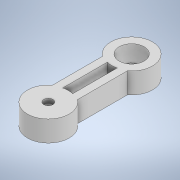
# Autodesk Inventor part: ramię_korby
Saved by Autodesk Inventor 2020 (Build 240168000, 168)
## iProperties
Created: 2020-08-09
Part Number: ramię_korby
Material: Aluminum 6061
Document SubType Name: Modeling
Designer: Hesekiel
Density: 2.7 g/cm^3
Appearance: Aluminum - Flat
Author: Hesekiel
Autodesk Inventor part; units mm, degrees
ref_plane "YZ Plane" through (0, 0, 0) normal (1, 0, 0) x (0, 1, 0)
ref_plane "XZ Plane" through (0, 0, 0) normal (0, 1, 0) x (-1, 0, 0)
ref_plane "XY Plane" through (0, 0, 0) normal (0, 0, 1) x (1, 0, 0)
sketch "Sketch1" plane through (0, 0, 0) normal (0, 1, 0) x (-1, 0, 0)
  circle A0 centre (0, 0) radius 15
  line L0 (15, 0) -> (-15, 0)
  line L1 (-15, 0) -> (-15, -100)
  line L2 (-15, -100) -> (15, -100)
  line L3 (15, -100) -> (15, 0)
  circle A1 centre (0, -100) radius 15
  circle A2 centre (0, 0) radius 25
  circle A3 centre (0, -100) radius 25
  point P0 (-15, -20)
  point P1 (-15, -80)
  point P2 (15, -80)
  point P3 (15, -20)
  dimension "d0" = 30
  dimension "d1" = 30
  dimension "d2" = 100
  dimension "d3" = 30
  dimension "d4" = 50
  dimension "d5" = 50
  constraints: 8 end point, 3 centre point, 3 coincident, 2 parallel, 1 horizontal, 1 horizontal alignment, 1 midpoint, 1 perpendicular, 2 other
  measures "d1" distance of L2.end L1.end
  measures "d2" distance of L1.end L0.end
  measures "d3" diameter of A1
  measures "d4" diameter of A2
  measures "d5" diameter of A3
extrude "Extrusion1" add sketch "Sketch1" along normal blind 15 contours L3 A2 L1 A0 | A0 L1 A2 L3 | L3 A3 L1 A2 | A3 L1 A1 L3 | L3 A1 L1 A3
shell "Shell1" thickness 9 removed faces 1 at (5, 15, -40)
sketch "Sketch2" plane through (0, 9, 0) normal (0, 1, 0) x (1, 0, 0)
  line L0 (-6, 76.7621) -> (-6, 23.2379) projected
  arc A0 (6, 23.2379) -> (-6, 23.2379) centre (0, 0) ccw projected
  line L1 (6, 23.2379) -> (6, 76.7621) projected
  arc A1 (-6, 76.7621) -> (6, 76.7621) centre (0, 100) ccw projected
extrude "Extrusion2" cut sketch "Sketch2" against normal blind 73.75
sketch "Sketch3" plane through (0, 0, 0) normal (0, -1, 0) x (1, 0, 0)
  line L0 (-6, -76.7621) -> (-6, -23.2379) projected
  arc A0 (-6, -23.2379) -> (6, -23.2379) centre (0, 0) ccw projected
  line L1 (6, -23.2379) -> (6, -76.7621) projected
  arc A1 (6, -76.7621) -> (-6, -76.7621) centre (0, -100) ccw projected
  arc A2 (-15, -80) -> (15, -80) centre (0, -100) ccw projected
  line L2 (15, -20) -> (15, -80) projected
  arc A3 (15, -20) -> (-15, -20) centre (0, 0) ccw projected
  line L3 (-15, -80) -> (-15, -20) projected
  circle A4 centre (0, 0) radius 15 projected
  circle A5 centre (0, -100) radius 15 projected
extrude "Extrusion3" add sketch "Sketch3" along normal blind 10
sketch "Sketch4" plane through (0, 15, 0) normal (0, 1, 0) x (1, 0, 0)
  circle A0 centre (0, 0) radius 15
  constraints: 1 centre point, 1 coincident
extrude "Extrusion4" add sketch "Sketch4" against normal blind 5
sketch "Sketch5" plane through (0, 15, 0) normal (0, 1, 0) x (1, 0, 0)
  circle A0 centre (0, 0) radius 5.5
  dimension "d15" = 11
  constraints: 1 centre point, 1 coincident
  measures "d15" diameter of A0
extrude "Extrusion5" cut sketch "Sketch5" against normal blind 89
sketch "Sketch6" plane through (0, -10, 0) normal (0, -1, 0) x (1, 0, 0)
  arc A0 (15, -20) -> (-15, -20) centre (0, 0) ccw projected
  line L0 (-15, -20) -> (-15, -80) projected
  arc A1 (-15, -80) -> (15, -80) centre (0, -100) ccw projected
  line L1 (15, -80) -> (15, -20) projected
  arc A2 (-6, -23.2379) -> (6, -23.2379) centre (0, 0) ccw projected
  line L2 (6, -23.2379) -> (6, -76.7621) projected
  arc A3 (6, -76.7621) -> (-6, -76.7621) centre (0, -100) ccw projected
  line L3 (-6, -76.7621) -> (-6, -23.2379) projected
  circle A4 centre (0, 0) radius 15 projected
  circle A5 centre (0, -100) radius 15 projected
extrude "Extrusion6" add sketch "Sketch6" against normal blind 5 contours A5
sketch "Sketch7" plane through (0, -10, 0) normal (0, -1, 0) x (1, 0, 0)
  arc A0 (15, -20) -> (-15, -20) centre (0, 0) ccw projected
  line L0 (-15, -20) -> (-15, -80) projected
  arc A1 (-15, -80) -> (15, -80) centre (0, -100) ccw projected
  line L1 (15, -80) -> (15, -20) projected
  arc A2 (-6, -23.2379) -> (6, -23.2379) centre (0, 0) ccw projected
  line L2 (6, -23.2379) -> (6, -76.7621) projected
  arc A3 (6, -76.7621) -> (-6, -76.7621) centre (0, -100) ccw projected
  line L3 (-6, -76.7621) -> (-6, -23.2379) projected
  circle A4 centre (0, 0) radius 15 projected
  circle A5 centre (0, -100) radius 15 projected
  circle A6 centre (0, -100) radius 5.5
  dimension "d20" = 11
  constraints: 1 centre point, 1 coincident
  measures "d20" diameter of A6
extrude "Extrusion7" cut sketch "Sketch7" against normal blind 115 contours A6
body "Solid1"
